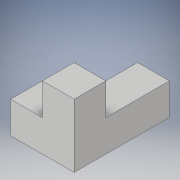
# Autodesk Inventor part: Additive Method(1)
Saved by Autodesk Inventor 2019 (Build 230136000, 136)
## iProperties
Created: 2019-09-05
Part Number: Additive Method(1)
Material: Generic
Document SubType Name: Modeling
Designer: IED8
Density: 1 g/cm^3
Appearance: Default
Author: IED8
Autodesk Inventor part; units mm, degrees
ref_plane "YZ Plane" through (0, 0, 0) normal (1, 0, 0) x (0, 1, 0)
ref_plane "XZ Plane" through (0, 0, 0) normal (0, 1, 0) x (-1, 0, 0)
ref_plane "XY Plane" through (0, 0, 0) normal (0, 0, 1) x (1, 0, 0)
sketch "Sketch1" plane through (0, 0, 0) normal (0, 1, 0) x (-1, 0, 0)
  line L0 (7.6204, 7.8637) -> (-30.4796, 7.8637)
  line L1 (-30.4796, 7.8637) -> (-30.4796, -49.2863)
  line L2 (-30.4796, -49.2863) -> (-11.4296, -49.2863)
  line L3 (-11.4296, -49.2863) -> (-11.4296, -30.2363)
  line L4 (-11.4296, -30.2363) -> (7.6204, -30.2363)
  line L5 (7.6204, -30.2363) -> (7.6204, 7.8637)
  point P0 (0, 0)
  dimension "d0" = 38.1
  dimension "d1" = 57.15
  dimension "d2" = 19.05
  dimension "d3" = 19.05
  dimension "d4" = 19.05
  constraints: 12 end point, 4 perpendicular, 1 horizontal
  measures "d0" distance of L0.start L0.end
  measures "d1" distance of L0.end L1.end
  measures "d2" distance of L1.end L2.end
  measures "d3" distance of L2.end L3.end
  measures "d4" distance of L3.end L4.end
extrude "Extrusion1" add sketch "Sketch1" along normal blind 19.05
sketch "Sketch2" plane through (0, 19.05, 0) normal (0, 1, 0) x (1, 0, 0)
  line L0 (11.4296, 11.1711) -> (11.4296, -7.8637)
  line L1 (-7.6204, -7.8637) -> (30.4796, -7.8637) projected
  line L2 (11.4296, 11.1711) -> (30.4796, 11.1711)
  line L3 (30.4796, -7.8637) -> (30.4796, 49.2863) projected
  line L4 (30.4796, 11.1711) -> (30.4796, -7.8637)
  line L5 (30.4796, -7.8637) -> (11.4296, -7.8637)
  point P0 (0, 0)
  constraints: 8 end point, 1 collinear, 1 horizontal, 1 midpoint, 1 perpendicular
extrude "Extrusion2" add sketch "Sketch2" along normal blind 19.05
body "Solid1"
